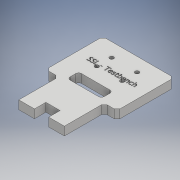
# Autodesk Inventor part: Support_Carte
Saved by Autodesk Inventor 2017 (Build 210142000, 142)
## iProperties
Part Number: Support_Carte
Material: Générique
Document SubType Name: Modeling
Designer: Darren
Density: 1 g/cm^3
Appearance: Par défaut
Author: Darren
Autodesk Inventor part; units mm, degrees
ref_plane "YZ Plane" through (0, 0, 0) normal (1, 0, 0) x (0, 1, 0)
ref_plane "XZ Plane" through (0, 0, 0) normal (0, 1, 0) x (-1, 0, 0)
ref_plane "XY Plane" through (0, 0, 0) normal (0, 0, 1) x (1, 0, 0)
sketch "Esquisse1" plane through (0, 0, 0) normal (0, 0, 1) x (1, 0, 0)
  line L0 (0, 0) -> (22, 0) construction
  line L1 (22, 0) -> (22, 27.9) construction
  line L2 (22, 27.9) -> (0, 27.9) construction
  line L3 (0, 27.9) -> (0, 0) construction
  line L4 (2, 25.9) -> (19.8, 25.9) construction
  line L5 (19.8, 25.9) -> (19.8, 15.4) construction
  line L6 (19.8, 15.4) -> (2, 15.4) construction
  line L7 (2, 15.4) -> (2, 25.9) construction
  circle A0 centre (2, 25.9) radius 1.4
  circle A1 centre (19.8, 25.9) radius 1.4
  circle A2 centre (19.8, 15.4) radius 1.4
  circle A3 centre (2, 15.4) radius 1.4
  line L8 (0, 0) -> (22, 0) construction
  line L9 (7.5, 23.15) -> (14.5, 23.15) construction
  line L10 (14.5, 23.15) -> (14.5, 18.15) construction
  line L11 (14.5, 18.15) -> (7.5, 18.15) construction
  line L12 (7.5, 18.15) -> (7.5, 23.15) construction
  line L13 (2, 25.9) -> (19.8, 15.4) construction
  line L14 (19.8, 25.9) -> (2, 15.4) construction
  line L15 (10.9, 20.65) -> (36, 20.65) construction
  line L16 (10.9, 20.65) -> (36, 20.65) construction
  line L17 (36, 20.65) -> (-14, 20.65) construction
  line L18 (-14, 33.65) -> (-14, -2.35)
  line L19 (36, -4.35) -> (36, 33.65)
  line L20 (10.9, 20.65) -> (10.9, 40.65) construction
  line L21 (10.9, 20.65) -> (36, 20.65) construction
  line L22 (-14, 20.65) -> (36, 20.65) construction
  line L23 (36, -2.35) -> (36, 33.65)
  line L24 (34, 35.65) -> (-12, 35.65)
  line L25 (-14, 33.65) -> (-14, -4.35)
  line L26 (-14, 33.65) -> (-12, 35.65)
  line L27 (34, 35.65) -> (36, 33.65)
  line L28 (16, -32.35) -> (16, -24.35)
  line L29 (16, -24.35) -> (6, -24.35)
  line L30 (6, -24.35) -> (6, -32.35)
  line L31 (-5, -32.35) -> (6, -32.35)
  line L32 (16, -32.35) -> (27, -32.35)
  line L33 (-5, -32.35) -> (-5, -6.35)
  line L34 (-7, -4.35) -> (-12, -4.35)
  line L35 (27, -32.35) -> (27, -6.35)
  line L36 (29, -4.35) -> (34, -4.35)
  line L37 (-14, -2.35) -> (-12, -4.35)
  line L38 (34, -4.35) -> (36, -2.35)
  line L39 (29, -4.35) -> (27, -6.35)
  line L40 (-7, -4.35) -> (-5, -6.35)
  point P0 (-5, -4.35)
  point P1 (27, -4.35)
  dimension "d0" = 22
  dimension "d1" = 27.9
  dimension "d2" = 17.8
  dimension "d3" = 10.5
  dimension "d4" = 2
  dimension "d5" = 2
  dimension "d6" = 2.8
  dimension "d7" = 2.8
  dimension "d8" = 2.8
  dimension "d9" = 2.8
  dimension "d12" = 7
  dimension "d13" = 5
  dimension "d15" = 7.5
  dimension "d16" = 2.75
  dimension "d18" = 0
  dimension "d21" = 20
  dimension "d22" = 90
  dimension "d36" = 2
  dimension "d37" = 2
  dimension "d38" = 2
  dimension "d39" = 2
  dimension "d50" = 15
  dimension "d66" = 25.1
  dimension "d67" = 50
  dimension "d68" = 9
  dimension "d69" = 32
  dimension "d70" = 11
  dimension "d71" = 11
  dimension "d72" = 25
  dimension "d73" = 8
  dimension "d74" = 8
  dimension "d75" = 28
  dimension "d76" = 25
  dimension "d77" = 2
  dimension "d78" = 2
  dimension "d79" = 2
  dimension "d80" = 2
  dimension "d81" = 2
  dimension "d82" = 2
  dimension "d83" = 2
  dimension "d84" = 2
  constraints: 82 end point, 12 parallel, 12 point on line, 9 horizontal, 6 perpendicular, 4 centre point, 4 coincident, 1 midpoint
  measures "d0" distance of L2.end L1.end
  measures "d1" distance of L1.end L0.end
  measures "d2" distance of L5.end L6.end
  measures "d3" distance of L4.end L5.end
  measures "d4" distance between parallel lines of L3 L7
  measures "d5" distance between parallel lines of L2 L4
  measures "d6" diameter of A0
  measures "d7" diameter of A1
  measures "d8" diameter of A2
  measures "d9" diameter of A3
  measures "d12" distance of L10.end L11.end
  measures "d13" distance of L9.end L10.end
  measures "d15" distance between parallel lines of L3 L12
  measures "d16" distance between parallel lines of L4 L9
  measures "d18" distance between parallel lines of L15 L16
  measures "d21" distance of L15.start L20.end
  measures "d22" angle of L21 L20
  measures "d36" horizontal distance of L24.start L19.end
  measures "d37" horizontal distance of L24.start L19.end
  measures "d38" horizontal distance of L18.start L24.end
  measures "d39" horizontal distance of L18.start L24.end
  measures "d50" distance between parallel lines of L24 L17
  measures "d66" distance between parallel lines of L23 L20
  measures "d67" distance between parallel lines of L19 L18
  measures "d68" distance between parallel lines of L33 L18
  measures "d69" distance between parallel lines of L35 L33
  measures "d70" distance between parallel lines of L33 L30
  measures "d71" distance between parallel lines of L35 L28
  measures "d72" distance between parallel lines of L34 L17
  measures "d73" distance between parallel lines of L29 L31
  measures "d74" distance between parallel lines of L32 L29
  measures "d75" distance between parallel lines of L32 L36
  measures "d76" distance between parallel lines of L17 L36
  measures "d77" distance of L18.end L25.end
  measures "d78" distance of L34.end L25.end
  measures "d79" distance of L36.end L19.start
  measures "d80" distance of L23.start L19.start
  measures "d81" distance of L36.start point (27, -4.35)
  measures "d82" distance of L35.end point (27, -4.35)
  measures "d83" distance of L34.start point (-5, -4.35)
  measures "d84" distance of L33.end point (-5, -4.35)
extrude "Extrusion1" add sketch "Esquisse1" along normal blind 6
sketch "Esquisse2" plane through (0, 0, 6) normal (0, 0, 1) x (1, 0, 0)
  line L0 (-9, 22.65) -> (31, 22.65) construction
  line L1 (31, 22.65) -> (31, 12.65) construction
  line L2 (31, 12.65) -> (-9, 12.65) construction
  line L3 (-9, 12.65) -> (-9, 22.65) construction
  circle A0 centre (2, 15.4) radius 1.4 construction
  circle A1 centre (19.8, 15.4) radius 1.4 construction
  circle A2 centre (19.8, 25.9) radius 1.4 construction
  circle A3 centre (2, 25.9) radius 1.4 construction
  line L4 (-14, 33.65) -> (-14, -2.35) construction
  line L5 (-5, -32.35) -> (6, -32.35) construction
  line L6 (6, -32.35) -> (6, -24.35) construction
  line L7 (6, -24.35) -> (16, -24.35) construction
  line L8 (16, -24.35) -> (16, -32.35) construction
  line L9 (16, -32.35) -> (27, -32.35) construction
  line L10 (36, 33.65) -> (34, 35.65) construction
  line L11 (34, 35.65) -> (-12, 35.65) construction
  line L12 (-12, 35.65) -> (-14, 33.65) construction
  line L13 (-12, -4.35) -> (-7, -4.35) projected
  line L14 (-5, -6.35) -> (-5, -32.35) projected
  line L15 (27, -32.35) -> (27, -6.35) projected
  line L16 (29, -4.35) -> (34, -4.35) projected
  line L17 (-14, -2.35) -> (-12, -4.35) projected
  line L18 (-7, -4.35) -> (-5, -6.35) projected
  line L19 (27, -6.35) -> (29, -4.35) projected
  line L20 (34, -4.35) -> (36, -2.35) projected
  line L21 (36, -2.35) -> (36, 33.65) projected
  line L22 (-5.8296, 16.056) -> (-5.6572, 16.4911)
  spline S0 degree 2 poles (-5.6572, 16.4911) (-5.5258, 16.3953) (-5.1317, 16.264) (-4.9758, 16.264) knots 0 0 0 1 2 2 2
  spline S1 degree 2 poles (-4.9758, 16.264) (-4.6994, 16.264) (-4.3655, 16.565) (-4.3655, 16.8003) knots 0 0 0 1 2 2 2
  spline S2 degree 2 poles (-4.3655, 16.8003) (-4.3655, 16.9727) (-4.5516, 17.2737) (-4.9265, 17.4489) knots 0 0 0 1 2 2 2
  line L23 (-4.9265, 17.4489) -> (-5.2029, 17.5802)
  spline S3 degree 2 poles (-5.2029, 17.5802) (-5.5586, 17.7444) (-5.8378, 18.1959) (-5.8378, 18.5161) knots 0 0 0 1 2 2 2
  spline S4 degree 2 poles (-5.8378, 18.5161) (-5.8378, 18.902) (-5.2905, 19.4109) (-4.8636, 19.4109) knots 0 0 0 1 2 2 2
  spline S5 degree 2 poles (-4.8636, 19.4109) (-4.2916, 19.4109) (-4.0672, 19.2249) knots 0 0 0 1 1 1
  line L24 (-4.0672, 19.2249) -> (-4.2068, 18.8144)
  spline S6 degree 2 poles (-4.2068, 18.8144) (-4.2998, 18.8828) (-4.6857, 19.0114) (-4.8526, 19.0114) knots 0 0 0 1 2 2 2
  spline S7 degree 2 poles (-4.8526, 19.0114) (-5.0907, 19.0114) (-5.3671, 18.7378) (-5.3671, 18.5243) knots 0 0 0 1 2 2 2
  spline S8 degree 2 poles (-5.3671, 18.5243) (-5.3671, 18.3902) (-5.2686, 18.174) (-5.0907, 18.0263) (-4.817, 17.8949) knots 0 0 0 1 2 3 3 3
  line L25 (-4.817, 17.8949) -> (-4.5352, 17.7608)
  spline S9 degree 2 poles (-4.5352, 17.7608) (-4.1822, 17.5939) (-3.8976, 17.1287) (-3.8976, 16.7702) knots 0 0 0 1 2 2 2
  spline S10 degree 2 poles (-3.8976, 16.7702) (-3.8976, 16.3816) (-4.5215, 15.8398) (-5.0442, 15.8398) knots 0 0 0 1 2 2 2
  spline S11 degree 2 poles (-5.0442, 15.8398) (-5.5039, 15.8398) (-5.8296, 16.056) knots 0 0 0 1 1 1
  line L26 (-3.509, 16.056) -> (-3.3366, 16.4911)
  spline S12 degree 2 poles (-3.3366, 16.4911) (-3.2052, 16.3953) (-2.8112, 16.264) (-2.6552, 16.264) knots 0 0 0 1 2 2 2
  spline S13 degree 2 poles (-2.6552, 16.264) (-2.3788, 16.264) (-2.045, 16.565) (-2.045, 16.8003) knots 0 0 0 1 2 2 2
  spline S14 degree 2 poles (-2.045, 16.8003) (-2.045, 16.9727) (-2.231, 17.2737) (-2.6059, 17.4489) knots 0 0 0 1 2 2 2
  line L27 (-2.6059, 17.4489) -> (-2.8823, 17.5802)
  spline S15 degree 2 poles (-2.8823, 17.5802) (-3.2381, 17.7444) (-3.5172, 18.1959) (-3.5172, 18.5161) knots 0 0 0 1 2 2 2
  spline S16 degree 2 poles (-3.5172, 18.5161) (-3.5172, 18.902) (-2.9699, 19.4109) (-2.543, 19.4109) knots 0 0 0 1 2 2 2
  spline S17 degree 2 poles (-2.543, 19.4109) (-1.9711, 19.4109) (-1.7467, 19.2249) knots 0 0 0 1 1 1
  line L28 (-1.7467, 19.2249) -> (-1.8862, 18.8144)
  spline S18 degree 2 poles (-1.8862, 18.8144) (-1.9793, 18.8828) (-2.3651, 19.0114) (-2.5321, 19.0114) knots 0 0 0 1 2 2 2
  spline S19 degree 2 poles (-2.5321, 19.0114) (-2.7701, 19.0114) (-3.0465, 18.7378) (-3.0465, 18.5243) knots 0 0 0 1 2 2 2
  spline S20 degree 2 poles (-3.0465, 18.5243) (-3.0465, 18.3902) (-2.948, 18.174) (-2.7701, 18.0263) (-2.4965, 17.8949) knots 0 0 0 1 2 3 3 3
  line L29 (-2.4965, 17.8949) -> (-2.2146, 17.7608)
  spline S21 degree 2 poles (-2.2146, 17.7608) (-1.8616, 17.5939) (-1.577, 17.1287) (-1.577, 16.7702) knots 0 0 0 1 2 2 2
  spline S22 degree 2 poles (-1.577, 16.7702) (-1.577, 16.3816) (-2.2009, 15.8398) (-2.7236, 15.8398) knots 0 0 0 1 2 2 2
  spline S23 degree 2 poles (-2.7236, 15.8398) (-3.1833, 15.8398) (-3.509, 16.056) knots 0 0 0 1 1 1
  line L30 (-1.0324, 15.9) -> (-1.0324, 19.3535)
  line L31 (-1.0324, 19.3535) -> (-0.5618, 19.3535)
  line L32 (-0.5618, 19.3535) -> (-0.5618, 16.3242)
  line L33 (-0.5618, 16.3242) -> (0.998, 16.3242)
  line L34 (0.998, 16.3242) -> (0.998, 15.9)
  line L35 (0.998, 15.9) -> (-1.0324, 15.9)
  line L36 (2.8862, 17.0931) -> (2.8862, 17.5063)
  line L37 (2.8862, 17.5063) -> (3.896, 17.5063)
  line L38 (3.896, 17.5063) -> (3.896, 17.0931)
  line L39 (3.896, 17.0931) -> (2.8862, 17.0931)
  line L40 (7.3495, 18.9293) -> (7.3495, 15.9)
  line L41 (7.3495, 15.9) -> (6.8788, 15.9)
  line L42 (6.8788, 15.9) -> (6.8788, 18.9293)
  line L43 (6.8788, 18.9293) -> (5.7815, 18.9293)
  line L44 (5.7815, 18.9293) -> (5.7815, 19.3535)
  line L45 (5.7815, 19.3535) -> (8.4961, 19.3535)
  line L46 (8.4961, 19.3535) -> (8.4961, 18.9293)
  line L47 (8.4961, 18.9293) -> (7.3495, 18.9293)
  line L48 (10.9836, 17.1205) -> (9.1638, 17.1205)
  spline S24 degree 2 poles (9.1638, 17.1205) (9.1638, 16.6772) (9.4073, 16.4391) knots 0 0 0 1 1 1
  spline S25 degree 2 poles (9.4073, 16.4391) (9.6208, 16.2311) (9.9601, 16.2311) knots 0 0 0 1 1 1
  spline S26 degree 2 poles (9.9601, 16.2311) (10.3432, 16.2311) (10.6005, 16.4555) knots 0 0 0 1 1 1
  line L49 (10.6005, 16.4555) -> (10.7893, 16.1326)
  spline S27 degree 2 poles (10.7893, 16.1326) (10.6853, 16.0286) (10.4719, 15.952) knots 0 0 0 1 1 1
  spline S28 degree 2 poles (10.4719, 15.952) (10.2009, 15.8535) (9.8726, 15.8535) knots 0 0 0 1 1 1
  spline S29 degree 2 poles (9.8726, 15.8535) (9.3964, 15.8535) (9.0625, 16.1764) knots 0 0 0 1 1 1
  spline S30 degree 2 poles (9.0625, 16.1764) (8.6931, 16.5321) (8.6931, 17.1342) knots 0 0 0 1 1 1
  spline S31 degree 2 poles (8.6931, 17.1342) (8.6931, 17.7581) (9.0735, 18.1357) knots 0 0 0 1 1 1
  spline S32 degree 2 poles (9.0735, 18.1357) (9.4128, 18.4723) (9.8753, 18.4723) knots 0 0 0 1 1 1
  spline S33 degree 2 poles (9.8753, 18.4723) (10.4171, 18.4723) (10.7209, 18.1686) knots 0 0 0 1 1 1
  spline S34 degree 2 poles (10.7209, 18.1686) (11.0192, 17.8758) (11.0192, 17.3941) knots 0 0 0 1 1 1
  spline S35 degree 2 poles (11.0192, 17.3941) (11.0192, 17.2464) (10.9836, 17.1205) knots 0 0 0 1 1 1
  spline S36 degree 2 poles (9.8972, 18.0947) (9.5989, 18.0947) (9.3964, 17.9031) knots 0 0 0 1 1 1
  spline S37 degree 2 poles (9.3964, 17.9031) (9.2021, 17.7198) (9.1775, 17.4461) knots 0 0 0 1 1 1
  line L50 (9.1775, 17.4461) -> (10.5731, 17.4461)
  spline S38 degree 2 poles (10.5731, 17.4461) (10.5731, 17.717) (10.4034, 17.8977) knots 0 0 0 1 1 1
  spline S39 degree 2 poles (10.4034, 17.8977) (10.2174, 18.0947) (9.8972, 18.0947) knots 0 0 0 1 1 1
  line L51 (11.3256, 16.0505) -> (11.4844, 16.4747)
  spline S40 degree 2 poles (11.4844, 16.4747) (11.8593, 16.2311) (12.0864, 16.2311) knots 0 0 0 1 1 1
  spline S41 degree 2 poles (12.0864, 16.2311) (12.5023, 16.2311) (12.5023, 16.5787) knots 0 0 0 1 1 1
  spline S42 degree 2 poles (12.5023, 16.5787) (12.5023, 16.8304) (12.1028, 17.0083) knots 0 0 0 1 1 1
  spline S43 degree 2 poles (12.1028, 17.0083) (11.7936, 17.1506) (11.5774, 17.2956) (11.4187, 17.4817) (11.3421, 17.6924) (11.3421, 17.8128) knots 0 0 0 1 2 3 4 4 4
  spline S44 degree 2 poles (11.3421, 17.8128) (11.3421, 18.1248) (11.7936, 18.4723) (12.1603, 18.4723) knots 0 0 0 1 2 2 2
  spline S45 degree 2 poles (12.1603, 18.4723) (12.4367, 18.4723) (12.8554, 18.2972) knots 0 0 0 1 1 1
  line L52 (12.8554, 18.2972) -> (12.7267, 17.884)
  spline S46 degree 2 poles (12.7267, 17.884) (12.4613, 18.0947) (12.1931, 18.0947) knots 0 0 0 1 1 1
  spline S47 degree 2 poles (12.1931, 18.0947) (12.0317, 18.0947) (11.8127, 17.9442) (11.8127, 17.8292) knots 0 0 0 1 2 2 2
  spline S48 degree 2 poles (11.8127, 17.8292) (11.8127, 17.5857) (12.0891, 17.4598) knots 0 0 0 1 1 1
  line L53 (12.0891, 17.4598) -> (12.4093, 17.3148)
  spline S49 degree 2 poles (12.4093, 17.3148) (12.7048, 17.1807) (12.973, 16.8359) (12.973, 16.5759) knots 0 0 0 1 2 2 2
  spline S50 degree 2 poles (12.973, 16.5759) (12.973, 16.2366) (12.4969, 15.8535) (12.0754, 15.8535) knots 0 0 0 1 2 2 2
  spline S51 degree 2 poles (12.0754, 15.8535) (11.6759, 15.8535) (11.3256, 16.0505) knots 0 0 0 1 1 1
  line L54 (13.6052, 18.0701) -> (13.3124, 18.0701)
  line L55 (13.3124, 18.0701) -> (13.3124, 18.4231)
  line L56 (13.3124, 18.4231) -> (13.6052, 18.4231)
  line L57 (13.6052, 18.4231) -> (13.6052, 18.9512)
  line L58 (13.6052, 18.9512) -> (14.0539, 19.1236)
  line L59 (14.0539, 19.1236) -> (14.0539, 18.4231)
  line L60 (14.0539, 18.4231) -> (14.7463, 18.4231)
  line L61 (14.7463, 18.4231) -> (14.7463, 18.0701)
  line L62 (14.7463, 18.0701) -> (14.0539, 18.0701)
  line L63 (14.0539, 18.0701) -> (14.0539, 16.8167)
  spline S52 degree 2 poles (14.0539, 16.8167) (14.0539, 16.4993) (14.2674, 16.2311) (14.5055, 16.2311) knots 0 0 0 1 2 2 2
  spline S53 degree 2 poles (14.5055, 16.2311) (14.6779, 16.2311) (14.8612, 16.3187) knots 0 0 0 1 1 1
  line L64 (14.8612, 16.3187) -> (14.9269, 15.9246)
  spline S54 degree 2 poles (14.9269, 15.9246) (14.6478, 15.8535) (14.3167, 15.8535) knots 0 0 0 1 1 1
  spline S55 degree 2 poles (14.3167, 15.8535) (14.0184, 15.8535) (13.6052, 16.2995) (13.6052, 16.6389) knots 0 0 0 1 2 2 2
  line L65 (13.6052, 16.6389) -> (13.6052, 18.0701)
  line L66 (15.7396, 16.0833) -> (15.5809, 15.8535)
  line L67 (15.5809, 15.8535) -> (15.3565, 15.8535)
  line L68 (15.3565, 15.8535) -> (15.3565, 19.4602)
  line L69 (15.3565, 19.4602) -> (15.8053, 19.4602)
  line L70 (15.8053, 19.4602) -> (15.8053, 18.2397)
  spline S56 degree 2 poles (15.8053, 18.2397) (15.8683, 18.3273) (16.2213, 18.4723) (16.3909, 18.4723) knots 0 0 0 1 2 2 2
  spline S57 degree 2 poles (16.3909, 18.4723) (16.9081, 18.4723) (17.5512, 17.7554) (17.5512, 17.2081) knots 0 0 0 1 2 2 2
  spline S58 degree 2 poles (17.5512, 17.2081) (17.5512, 16.5759) (16.9054, 15.8535) (16.3526, 15.8535) knots 0 0 0 1 2 2 2
  spline S59 degree 2 poles (16.3526, 15.8535) (16.1747, 15.8535) (15.8272, 15.9876) (15.7396, 16.0833) knots 0 0 0 1 2 2 2
  line L71 (15.8053, 17.8977) -> (15.8053, 16.4418)
  spline S60 degree 2 poles (15.8053, 16.4418) (15.8053, 16.4035) (16.1392, 16.2311) (16.2267, 16.2311) knots 0 0 0 1 2 2 2
  spline S61 degree 2 poles (16.2267, 16.2311) (16.6837, 16.2311) (17.0805, 16.669) (17.0805, 17.1862) knots 0 0 0 1 2 2 2
  spline S62 degree 2 poles (17.0805, 17.1862) (17.0805, 17.6131) (16.6181, 18.0947) (16.2267, 18.0947) knots 0 0 0 1 2 2 2
  spline S63 degree 2 poles (16.2267, 18.0947) (16.1446, 18.0947) (15.8491, 17.9524) (15.8053, 17.8977) knots 0 0 0 1 2 2 2
  line L72 (20.1728, 17.1205) -> (18.353, 17.1205)
  spline S64 degree 2 poles (18.353, 17.1205) (18.353, 16.6772) (18.5966, 16.4391) knots 0 0 0 1 1 1
  spline S65 degree 2 poles (18.5966, 16.4391) (18.81, 16.2311) (19.1493, 16.2311) knots 0 0 0 1 1 1
  spline S66 degree 2 poles (19.1493, 16.2311) (19.5324, 16.2311) (19.7897, 16.4555) knots 0 0 0 1 1 1
  line L73 (19.7897, 16.4555) -> (19.9785, 16.1326)
  spline S67 degree 2 poles (19.9785, 16.1326) (19.8745, 16.0286) (19.6611, 15.952) knots 0 0 0 1 1 1
  spline S68 degree 2 poles (19.6611, 15.952) (19.3901, 15.8535) (19.0618, 15.8535) knots 0 0 0 1 1 1
  spline S69 degree 2 poles (19.0618, 15.8535) (18.5856, 15.8535) (18.2518, 16.1764) knots 0 0 0 1 1 1
  spline S70 degree 2 poles (18.2518, 16.1764) (17.8823, 16.5321) (17.8823, 17.1342) knots 0 0 0 1 1 1
  spline S71 degree 2 poles (17.8823, 17.1342) (17.8823, 17.7581) (18.2627, 18.1357) knots 0 0 0 1 1 1
  spline S72 degree 2 poles (18.2627, 18.1357) (18.602, 18.4723) (19.0645, 18.4723) knots 0 0 0 1 1 1
  spline S73 degree 2 poles (19.0645, 18.4723) (19.6063, 18.4723) (19.9101, 18.1686) knots 0 0 0 1 1 1
  spline S74 degree 2 poles (19.9101, 18.1686) (20.2084, 17.8758) (20.2084, 17.3941) knots 0 0 0 1 1 1
  spline S75 degree 2 poles (20.2084, 17.3941) (20.2084, 17.2464) (20.1728, 17.1205) knots 0 0 0 1 1 1
  spline S76 degree 2 poles (19.0864, 18.0947) (18.7881, 18.0947) (18.5856, 17.9031) knots 0 0 0 1 1 1
  spline S77 degree 2 poles (18.5856, 17.9031) (18.3913, 17.7198) (18.3667, 17.4461) knots 0 0 0 1 1 1
  line L74 (18.3667, 17.4461) -> (19.7623, 17.4461)
  spline S78 degree 2 poles (19.7623, 17.4461) (19.7623, 17.717) (19.5926, 17.8977) knots 0 0 0 1 1 1
  spline S79 degree 2 poles (19.5926, 17.8977) (19.4066, 18.0947) (19.0864, 18.0947) knots 0 0 0 1 1 1
  line L75 (22.2334, 15.9) -> (22.2334, 17.3695)
  spline S80 degree 2 poles (22.2334, 17.3695) (22.2334, 17.7718) (21.9898, 18.0947) (21.7052, 18.0947) knots 0 0 0 1 2 2 2
  spline S81 degree 2 poles (21.7052, 18.0947) (21.552, 18.0947) (21.2181, 17.9113) (21.1278, 17.7772) knots 0 0 0 1 2 2 2
  line L76 (21.1278, 17.7772) -> (21.1278, 15.9)
  line L77 (21.1278, 15.9) -> (20.679, 15.9)
  line L78 (20.679, 15.9) -> (20.679, 18.4231)
  line L79 (20.679, 18.4231) -> (20.9855, 18.4231)
  line L80 (20.9855, 18.4231) -> (21.1278, 18.0974)
  spline S82 degree 2 poles (21.1278, 18.0974) (21.3495, 18.4723) (21.853, 18.4723) knots 0 0 0 1 1 1
  spline S83 degree 2 poles (21.853, 18.4723) (22.6822, 18.4723) (22.6822, 17.4625) knots 0 0 0 1 1 1
  line L81 (22.6822, 17.4625) -> (22.6822, 15.9)
  line L82 (22.6822, 15.9) -> (22.2334, 15.9)
  line L83 (25.2353, 18.2206) -> (25.0109, 17.9059)
  spline S84 degree 2 poles (25.0109, 17.9059) (24.9425, 17.9743) (24.5923, 18.0947) (24.4253, 18.0947) knots 0 0 0 1 2 2 2
  spline S85 degree 2 poles (24.4253, 18.0947) (24.0559, 18.0947) (23.6235, 17.583) (23.6235, 17.1369) knots 0 0 0 1 2 2 2
  spline S86 degree 2 poles (23.6235, 17.1369) (23.6235, 16.6963) (24.0614, 16.2311) (24.45, 16.2311) knots 0 0 0 1 2 2 2
  spline S87 degree 2 poles (24.45, 16.2311) (24.751, 16.2311) (25.0575, 16.4637) knots 0 0 0 1 1 1
  line L84 (25.0575, 16.4637) -> (25.2353, 16.0861)
  spline S88 degree 2 poles (25.2353, 16.0861) (24.8741, 15.8535) (24.3432, 15.8535) knots 0 0 0 1 1 1
  spline S89 degree 2 poles (24.3432, 15.8535) (23.826, 15.8535) (23.1529, 16.5458) (23.1529, 17.1369) knots 0 0 0 1 2 2 2
  spline S90 degree 2 poles (23.1529, 17.1369) (23.1529, 17.7417) (23.8561, 18.4723) (24.4691, 18.4723) knots 0 0 0 1 2 2 2
  spline S91 degree 2 poles (24.4691, 18.4723) (24.6661, 18.4723) (25.1259, 18.3081) (25.2353, 18.2206) knots 0 0 0 1 2 2 2
  line L85 (27.2604, 15.9) -> (27.2604, 17.4872)
  spline S92 degree 2 poles (27.2604, 17.4872) (27.2604, 17.769) (26.984, 18.0947) (26.7322, 18.0947) knots 0 0 0 1 2 2 2
  spline S93 degree 2 poles (26.7322, 18.0947) (26.568, 18.0947) (26.2424, 17.9031) (26.1548, 17.7772) knots 0 0 0 1 2 2 2
  line L86 (26.1548, 17.7772) -> (26.1548, 15.9)
  line L87 (26.1548, 15.9) -> (25.706, 15.9)
  line L88 (25.706, 15.9) -> (25.706, 19.4602)
  line L89 (25.706, 19.4602) -> (26.1548, 19.4602)
  line L90 (26.1548, 19.4602) -> (26.1548, 18.1467)
  spline S94 degree 2 poles (26.1548, 18.1467) (26.2451, 18.2862) (26.6419, 18.4723) (26.8554, 18.4723) knots 0 0 0 1 2 2 2
  spline S95 degree 2 poles (26.8554, 18.4723) (27.2549, 18.4723) (27.7091, 17.9442) (27.7091, 17.4872) knots 0 0 0 1 2 2 2
  line L91 (27.7091, 17.4872) -> (27.7091, 15.9)
  line L92 (27.7091, 15.9) -> (27.2604, 15.9)
  point P0 (0, 0)
  dimension "d56" = 40
  dimension "d57" = 5
  dimension "d58" = 45
  dimension "d59" = 10
  constraints: 2 other
  measures "d56" distance between parallel lines of L1 L3
  measures "d57" distance between parallel lines of L4 L3
  measures "d58" distance between parallel lines of L9 L2
  measures "d59" distance between parallel lines of L2 L0
emboss "Gravure1" sketch "Esquisse2" operation cut depth 1 direction (0, 0, -1)
ref_plane "Plan de construction1" through (2, 25.9, 0) normal (0.5080771, 0.8613116, 0) x (0, 0, 1)
ref_plane "Plan de construction2" through (2, 15.4, 0) normal (-0.5080771, 0.8613116, 0) x (0, 0, 1)
sketch "Esquisse3" plane through (0, 0, 6) normal (0, 0, 1) x (1, 0, 0)
  line L0 (-14, 33.65) -> (-14, -2.35) construction
  line L1 (-14, -2.35) -> (-12, -4.35) construction
  line L2 (-12, -4.35) -> (-7, -4.35) construction
  line L3 (-7, -4.35) -> (-5, -6.35) construction
  line L4 (-5, -6.35) -> (-5, -32.35) construction
  line L5 (-5, -32.35) -> (6, -32.35) construction
  line L6 (6, -32.35) -> (6, -24.35) construction
  line L7 (6, -24.35) -> (16, -24.35) construction
  line L8 (16, -24.35) -> (16, -32.35) construction
  line L9 (16, -32.35) -> (27, -32.35) construction
  line L10 (27, -32.35) -> (27, -6.35) construction
  line L11 (27, -6.35) -> (29, -4.35) construction
  line L12 (29, -4.35) -> (34, -4.35) construction
  line L13 (34, -4.35) -> (36, -2.35) construction
  line L14 (36, -2.35) -> (36, 33.65) construction
  line L15 (36, 33.65) -> (34, 35.65) construction
  line L16 (34, 35.65) -> (-12, 35.65) construction
  line L17 (-12, 35.65) -> (-14, 33.65) construction
  circle A0 centre (2, 25.9) radius 1.4 construction
  circle A1 centre (19.8, 25.9) radius 1.4 construction
  arc A2 (18.525, 15.9782) -> (21.1077, 15.9) centre (19.8, 15.4) ccw construction
  arc A3 (0.6923, 15.9) -> (0.9484, 16.3242) centre (2, 15.4) ccw construction
  line L18 (25.2353, 18.2206) -> (25.0109, 17.9059) construction
  line L19 (25.0575, 16.4637) -> (25.2353, 16.0861) construction
  line L20 (22.6822, 17.4625) -> (22.6822, 15.9) construction
  line L21 (22.6822, 15.9) -> (22.2334, 15.9) construction
  line L22 (22.2334, 15.9) -> (22.2334, 17.3695) construction
  line L23 (21.1278, 17.7772) -> (21.1278, 15.9) construction
  line L24 (21.1278, 15.9) -> (21.1077, 15.9) construction
  line L25 (20.679, 16.4896) -> (20.679, 18.4231) construction
  line L26 (20.679, 18.4231) -> (20.9855, 18.4231) construction
  line L27 (20.9855, 18.4231) -> (21.1278, 18.0974) construction
  line L28 (14.0539, 18.0701) -> (14.0539, 16.8167) construction
  line L29 (14.8612, 16.3187) -> (14.9269, 15.9246) construction
  line L30 (13.6052, 16.6389) -> (13.6052, 18.0701) construction
  line L31 (13.6052, 18.0701) -> (13.3124, 18.0701) construction
  line L32 (13.3124, 18.0701) -> (13.3124, 18.4231) construction
  line L33 (13.3124, 18.4231) -> (13.6052, 18.4231) construction
  line L34 (13.6052, 18.4231) -> (13.6052, 18.9512) construction
  line L35 (13.6052, 18.9512) -> (14.0539, 19.1236) construction
  line L36 (14.0539, 19.1236) -> (14.0539, 18.4231) construction
  line L37 (14.0539, 18.4231) -> (14.7463, 18.4231) construction
  line L38 (14.7463, 18.4231) -> (14.7463, 18.0701) construction
  line L39 (14.7463, 18.0701) -> (14.0539, 18.0701) construction
  line L40 (20.1728, 17.1205) -> (18.353, 17.1205) construction
  line L41 (5.7815, 19.3535) -> (8.4961, 19.3535) construction
  line L42 (8.4961, 19.3535) -> (8.4961, 18.9293) construction
  line L43 (8.4961, 18.9293) -> (7.3495, 18.9293) construction
  line L44 (7.3495, 18.9293) -> (7.3495, 15.9) construction
  line L45 (7.3495, 15.9) -> (6.8788, 15.9) construction
  line L46 (6.8788, 15.9) -> (6.8788, 18.9293) construction
  line L47 (6.8788, 18.9293) -> (5.7815, 18.9293) construction
  line L48 (5.7815, 18.9293) -> (5.7815, 19.3535) construction
  line L49 (15.7396, 16.0833) -> (15.5809, 15.8535) construction
  line L50 (15.5809, 15.8535) -> (15.3565, 15.8535) construction
  line L51 (15.3565, 15.8535) -> (15.3565, 19.4602) construction
  line L52 (15.3565, 19.4602) -> (15.8053, 19.4602) construction
  line L53 (15.8053, 19.4602) -> (15.8053, 18.2397) construction
  line L54 (0.6923, 15.9) -> (-1.0324, 15.9) construction
  line L55 (-1.0324, 15.9) -> (-1.0324, 19.3535) construction
  line L56 (-1.0324, 19.3535) -> (-0.5618, 19.3535) construction
  line L57 (-0.5618, 19.3535) -> (-0.5618, 16.3242) construction
  line L58 (-0.5618, 16.3242) -> (0.9484, 16.3242) construction
  line L59 (12.0891, 17.4598) -> (12.4093, 17.3148) construction
  line L60 (11.3256, 16.0505) -> (11.4844, 16.4747) construction
  line L61 (12.8554, 18.2972) -> (12.7267, 17.884) construction
  line L62 (-4.817, 17.8949) -> (-4.5352, 17.7608) construction
  line L63 (-5.8296, 16.056) -> (-5.6572, 16.4911) construction
  line L64 (-4.9265, 17.4489) -> (-5.2029, 17.5802) construction
  line L65 (-4.0672, 19.2249) -> (-4.2068, 18.8144) construction
  line L66 (10.9836, 17.1205) -> (9.1638, 17.1205) construction
  line L67 (10.6005, 16.4555) -> (10.7893, 16.1326) construction
  line L68 (-2.4965, 17.8949) -> (-2.2146, 17.7608) construction
  line L69 (-3.509, 16.056) -> (-3.3366, 16.4911) construction
  line L70 (-2.6059, 17.4489) -> (-2.8823, 17.5802) construction
  line L71 (-1.7467, 19.2249) -> (-1.8862, 18.8144) construction
  line L72 (2.8862, 17.0931) -> (2.8862, 17.5063) construction
  line L73 (2.8862, 17.5063) -> (3.896, 17.5063) construction
  line L74 (3.896, 17.5063) -> (3.896, 17.0931) construction
  line L75 (3.896, 17.0931) -> (2.8862, 17.0931) construction
  line L76 (27.7091, 17.4872) -> (27.7091, 15.9) construction
  line L77 (27.7091, 15.9) -> (27.2604, 15.9) construction
  line L78 (27.2604, 15.9) -> (27.2604, 17.4872) construction
  line L79 (26.1548, 17.7772) -> (26.1548, 15.9) construction
  line L80 (26.1548, 15.9) -> (25.706, 15.9) construction
  line L81 (25.706, 15.9) -> (25.706, 19.4602) construction
  line L82 (25.706, 19.4602) -> (26.1548, 19.4602) construction
  line L83 (26.1548, 19.4602) -> (26.1548, 18.1467) construction
  line L84 (1, 5.65) -> (21, 5.65)
  line L85 (23, 3.65) -> (23, -0.35)
  line L86 (21, -2.35) -> (1, -2.35)
  line L87 (-1, -0.35) -> (-1, 3.65)
  arc A4 (1, 5.65) -> (-1, 3.65) centre (1, 3.65) ccw
  arc A5 (-1, -0.35) -> (1, -2.35) centre (1, -0.35) ccw
  arc A6 (21, -2.35) -> (23, -0.35) centre (21, -0.35) ccw
  arc A7 (23, 3.65) -> (21, 5.65) centre (21, 3.65) ccw
  arc A8 (20.679, 16.4896) -> (18.7495, 16.3254) centre (19.8, 15.4) ccw projected
  point P0 (0, 0)
  point P1 (-1, 5.65)
  point P2 (23, -2.35)
  point P3 (23, 5.65)
  point P4 (-1, -2.35)
  dimension "d88" = 24
  dimension "d89" = 8
  dimension "d90" = 13
  dimension "d91" = 30
  dimension "d94" = 2
  constraints: 8 end point, 8 point on circle, 8 point on line, 8 tangent, 4 centre point, 3 equal radius, 2 parallel, 1 horizontal, 1 perpendicular, 81 other
  measures "d88" distance of point (23, -2.35) point (-1, -2.35)
  measures "d89" distance of point (23, 5.65) point (23, -2.35)
  measures "d90" distance between parallel lines of L14 L85
  measures "d91" distance between parallel lines of L16 L84
  measures "d94" radius of A4
extrude "Extrusion2" cut sketch "Esquisse3" against normal blind 10
equation "\"d78\" = d77"
equation "\"d79\" = d77"
equation "\"d80\" = d79"
equation "\"d81\" = d77"
equation "\"d82\" = d81"
equation "\"d83\" = d77"
equation "\"d84\" = d83"
